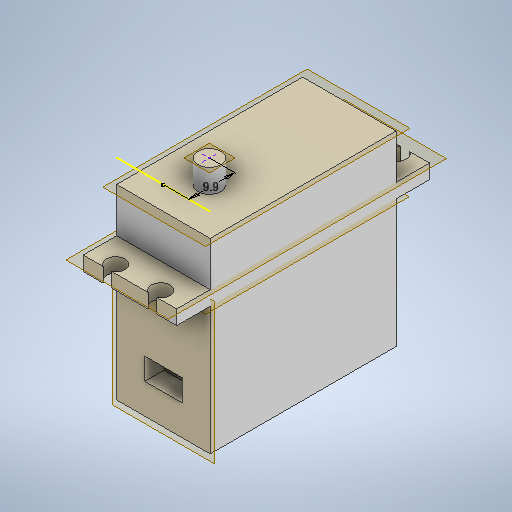
# Autodesk Inventor part: Part
Saved by Autodesk Inventor 2025.2 (Build 292293000, 293)
## iProperties
Created: 2024-12-14
Part Number: Part
Material: 一般
Document SubType Name: Modeling
Designer: mahhy
Density: 1 g/cm^3
Appearance: 既定
Author: mahhy
Autodesk Inventor part; units mm, degrees
ref_plane "YZ Plane" through (0, 0, 0) normal (1, 0, 0) x (0, 1, 0)
ref_plane "XZ Plane" through (0, 0, 0) normal (0, 1, 0) x (-1, 0, 0)
ref_plane "XY Plane" through (0, 0, 0) normal (0, 0, 1) x (1, 0, 0)
sketch "スケッチ2" plane through (0, 0, 0) normal (0, 1, 0) x (-1, 0, 0)
  line L0 (0, 0) -> (20.1, 0)
  line L1 (20.1, 0) -> (20.1, -40)
  line L2 (20.1, -40) -> (0, -40)
  line L3 (0, -40) -> (0, 0)
  dimension "d0" = 20.1
  dimension "d1" = 40
  constraints: 8 end point, 2 parallel, 1 horizontal, 1 perpendicular
  measures "d0" distance of L1.end L2.end
  measures "d1" distance of L0.end L1.end
extrude "押し出し1" add sketch "スケッチ2" along normal blind 27.5
ref_plane "作業平面1" through (0, 27.5, 0) normal (0, 1, 0) x (1, 0, 0)
sketch "スケッチ3" plane through (0, 27.5, 0) normal (0, 1, 0) x (1, 0, 0)
  line L0 (-20.1, 47.19) -> (0, 47.19)
  line L1 (0, 47.19) -> (0, -7.19)
  line L2 (0, -7.19) -> (-20.1, -7.19)
  line L3 (-20.1, -7.19) -> (-20.1, 47.19)
  line L4 (-20.1, 40) -> (-20.1, 0) projected
  line L5 (0, 40) -> (-20.1, 40) projected
  point P0 (0, 0)
  point P1 (-20.1, 20)
  point P2 (-20.1, 20)
  point P3 (-10.05, 47.19)
  point P4 (-10.05, 40)
  point P5 (-10.05, 40)
  point P6 (0, 40)
  point P7 (-20.1, 40)
  dimension "d5" = 20.1
  dimension "d6" = 54.38
  dimension "d7" = 0
  dimension "d8" = 0
  constraints: 8 end point, 5 midpoint, 2 parallel, 1 horizontal, 1 perpendicular
  measures "d5" distance of L1.end L2.end
  measures "d6" distance of L0.end L1.end
  measures "d7" distance of point (-20.1, 20) point (-20.1, 20)
  measures "d8" horizontal distance of point (-10.05, 40) point (-10.05, 47.19)
extrude "押し出し2" add sketch "スケッチ3" along normal blind 3.1
ref_plane "作業平面2" through (0, 30.6, 0) normal (0, 1, 0) x (1, 0, 0)
sketch "スケッチ4" plane through (0, 30.6, 0) normal (0, 1, 0) x (1, 0, 0)
  line L0 (0, -7.19) -> (0, 0) projected
  line L1 (0, 0) -> (-20.1, 0)
  line L2 (-20.1, 0) -> (-20.1, 40)
  line L3 (-20.1, 40) -> (0, 40)
  line L4 (0, 40) -> (0, 0)
  circle A0 centre (-14.9, 45.43) radius 2
  circle A1 centre (-5.2, 45.43) radius 2
  line L5 (-15.85, 47.19) -> (-13.95, 47.19)
  line L6 (-6.15, 47.19) -> (-4.25, 47.19)
  line L7 (-13.95, 47.19) -> (-6.15, 47.19)
  line L8 (0, 47.19) -> (-20.1, 47.19) projected
  point P0 (-10.05, 47.19)
  dimension "d12" = 40
  dimension "d23" = 4
  dimension "d24" = 4
  dimension "d27" = 1.9
  dimension "d28" = 1.9
  dimension "d29" = 7.8
  dimension "d53" = 20.1
  constraints: 14 end point, 4 point on circle, 3 coincident, 2 centre point, 2 collinear, 2 midpoint, 2 parallel, 1 horizontal, 1 perpendicular
  measures "d12" distance of L1.end L2.end
  measures "d23" diameter of A0
  measures "d24" diameter of A1
  measures "d27" distance of L5.start L5.end
  measures "d28" distance of L6.start L6.end
  measures "d29" distance of L6.start L7.start
  measures "d53" distance of L0.end L1.end
extrude "押し出し3" add sketch "スケッチ4" along normal blind 9.55 contours L1 L2 L3 L4
sketch "スケッチ7" plane through (0, 30.6, 0) normal (0, 1, 0) x (1, 0, 0)
  circle A0 centre (-14.9, 45.43) radius 2
  circle A1 centre (-5.2, 45.43) radius 2
  circle A2 centre (-14.9, -5.43) radius 2
  circle A3 centre (-5.2, -5.43) radius 2
  line L0 (-13.95, 47.19) -> (-15.85, 47.19)
  line L1 (-6.15, 47.19) -> (-4.25, 47.19)
  line L2 (-15.85, -7.19) -> (-13.95, -7.19)
  line L3 (-6.15, -7.19) -> (-4.25, -7.19)
  line L4 (-13.95, -7.19) -> (-6.15, -7.19)
  line L5 (-13.95, 47.19) -> (-6.15, 47.19)
  line L6 (0, 47.19) -> (-20.1, 47.19) projected
  line L7 (-20.1, -7.19) -> (0, -7.19) projected
  point P0 (0, 0)
  point P1 (-10.05, -7.19)
  point P2 (-10.05, 47.19)
  point P3 (-10.05, -7.19)
  dimension "d33" = 4
  dimension "d34" = 4
  dimension "d35" = 4
  dimension "d36" = 4
  dimension "d37" = 1.9
  dimension "d38" = 1.9
  dimension "d39" = 1.9
  dimension "d40" = 1.9
  dimension "d41" = 7.8
  dimension "d42" = 7.8
  constraints: 12 end point, 8 point on circle, 5 collinear, 5 midpoint, 4 centre point, 1 horizontal
  measures "d33" diameter of A0
  measures "d34" diameter of A1
  measures "d35" diameter of A2
  measures "d36" diameter of A3
  measures "d37" distance of L0.start L0.end
  measures "d38" distance of L1.start L1.end
  measures "d39" distance of L2.start L2.end
  measures "d40" distance of L3.start L3.end
  measures "d41" distance of L3.start L2.end
  measures "d42" distance of L0.start L1.start
extrude "押し出し6" cut sketch "スケッチ7" against normal through all contours A0 L0 | L1 A1 | A2 L2 | A3 L3 | L3 A3 | L2 A2 picked at (-15.3262, 45.9006) picked at (-5.6145, 46.6348)
ref_plane "作業平面5" through (-20.1, 0, 0) normal (0, 0, 1) x (1, 0, 0)
sketch "スケッチ8" plane through (-20.1, 0, 0) normal (0, 0, 1) x (1, 0, 0)
  line L0 (6.05, 11.2) -> (14.05, 11.2)
  line L1 (14.05, 11.2) -> (14.05, 6.5)
  line L2 (14.05, 6.5) -> (6.05, 6.5)
  line L3 (6.05, 6.5) -> (6.05, 11.2)
  line L4 (0, 0) -> (0, 27.5) projected
  line L5 (20.1, 0) -> (20.1, 27.5) projected
  line L6 (0, 0) -> (20.1, 0) projected
  dimension "d46" = 8
  dimension "d47" = 4.7
  dimension "d48" = 6.05
  dimension "d49" = 6.05
  dimension "d50" = 6.5
  constraints: 8 end point, 2 parallel, 1 horizontal, 1 perpendicular
  measures "d46" distance of L1.end L2.end
  measures "d47" distance of L0.end L1.end
  measures "d48" distance between parallel lines of L4 L3
  measures "d49" distance between parallel lines of L5 L1
  measures "d50" distance between parallel lines of L6 L2
extrude "押し出し7" cut sketch "スケッチ8" against normal blind 4.15
ref_plane "作業平面6" through (0, 40.15, 0) normal (0, 1, 0) x (1, 0, 0)
sketch "スケッチ10" plane through (0, 40.15, 0) normal (0, 1, 0) x (1, 0, 0)
  line L0 (-20.1, 0) -> (0, 0) projected
  circle A0 centre (-10.05, 9.9) radius 2.5
  point P0 (-10.05, 0)
  dimension "d57" = 9.9
  dimension "d59" = 5
  constraints: 1 centre point, 1 coincident, 1 midpoint
  measures "d57" distance from line of L0 point (-10.05, 9.9)
  measures "d59" diameter of A0
extrude "押し出し8" add sketch "スケッチ10" along normal blind 5
ref_plane "作業平面7" through (-10.05, 45.15, -9.9) normal (0, 1, 0) x (1, 0, 0)
sketch "スケッチ11" plane through (-10.05, 45.15, -9.9) normal (0, 1, 0) x (1, 0, 0)
  line L0 (-10.05, -9.9) -> (10.05, -9.9) projected
  point P0 (0, 0)
  point P1 (0, -9.9)
  dimension "d63" = 9.9
  constraints: 1 midpoint
  measures "d63" distance of point (0, 0) point (0, -9.9)
